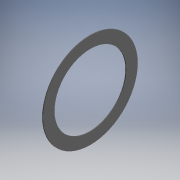
# Autodesk Inventor part: WA673SA Shield
Saved by Autodesk Inventor 2017.3 (Build 213256000, 256)
## iProperties
Part Number: WA673SA Shield
Material: Generic
Catalog Web Link: www.cadenas.de
Description: Six types s-Metric system sizes
Vendor: NTN
Document SubType Name: Modeling
Designer: partserver
Manufacturer: NTN
Mass: 0.00039028 g
Surface Area: 0.195934 cm^2
Volume: 0.00039028 cm^3
Density: 1 g/cm^3
Appearance: PSOLRGB-128-128-128
Category: PARTsolutions
Company: NTN
Title: WA673SA Shield
Author: Cadenas PARTsolutions
Comments: Metric system sizes
PSOL_IDENT_0: {$CADENAS_DATA\23d-libs\ntn\ball_roller_bearings\miniature_extra_small_bb\metric_system_sizes\mss_s.
PSOL_IDENT_1: prj},176 {VTYP=3D},{NB=WA673SA Shield},{LINA=WA673SA Shield},{NN=Six types s},{DATE=21.12.2021 04:23
PSOL_IDENT_2: :05},{GEOMDATE=06.03.2020 10:08:02},{VERSION=},{LINEID=11430},{WBVAR=},{WBNUMERIC=}  {NB=WA673SA Shi
PSOL_IDENT_3: eld},{LINA=WA673SA Shield},{KT=DUMMY},{IDNR=},{SD=3.0},{D=6},{B=2.0},{R=0.08},{ORDER=WA673SA},{CR=24
PSOL_IDENT_4: 2},{COR=94},{CRF=25},{CORF=9,5},{LSG=60 000},{LSO=71 000},{MASS=0.20},{ORDER1=673},{D1=7.2},{D2=7.2}
PSOL_IDENT_5: ,{C1=0.6},{C2=0.6},{WSS=WA673SA},{WDS=SSA},{UTWF=FL673},{FORSS=FLWA673SA},{FORDS=SSA},{DA1=3,6},{DA2=
PSOL_IDENT_6: 4,1},{DA=5,4},{RAS=0,08},{MASS1=0.26},{B1=2.5},{VERS=2},{X=1.5},{N=9},{O=14.13},{RB=0.444}
NB: WA673SA Shield
NN: Six types s
NT: Metric system sizes
NBSYN: $ORDER. Shield
LINA: WA673SA Shield
CATALOG: NTN Corporation
SD: 3
D: 6
B: 2
R: 0.08
CR: 242
COR: 94
CRF: 25
CORF: 9,5
LSG: 60 000
LSO: 71 000
MASS: 0.2
ORDER1: 673
D1: 7.2
D2: 7.2
C1: 0.6
C2: 0.6
WSS: WA673SA
WDS: SSA
UTWF: FL673
FORSS: FLWA673SA
FORDS: SSA
DA1: 3,6
DA2: 4,1
DA: 5,4
RAS: 0,08
MASS1: 0.26
B1: 2.5
VERS: 2
SUPPLIER: NTN
ARTICLENO: WA673SA Shield
BOMINFO: WA673SA Shield
CREATOR: CADENAS GmbH
Autodesk Inventor part; units mm, degrees
sketch "Sketch_1" plane through (0, 0, 0) normal (0, 0, 1) x (1, 0, 0)
  line L0 (-0.0138, 0) -> (-0.0563, 0)
  line L1 (-0.0563, 2.616) -> (-0.0563, 1.98)
  line L2 (-0.0563, 1.98) -> (-0.0138, 1.98)
  line L3 (-0.0138, 1.98) -> (-0.0138, 2.616)
  line L4 (-0.0138, 2.616) -> (-0.0563, 2.616)
  constraints: 10 end point
revolve "Revolution1" add sketch "Sketch_1" angle 360 about axis through (-0.0138, 0, 0) along (1, 0, 0)
ref_plane "mss_s_XY" through (0, 0, 0) normal (1, 0, 0) x (0, 0, -1)
ref_plane "mss_s_YZ" through (0, 0, 0) normal (0, 0, -1) x (0, 1, 0)
ref_plane "mss_s_ZX" through (0, 0, 0) normal (0, 1, 0) x (1, 0, 0)
body "Solid1"
